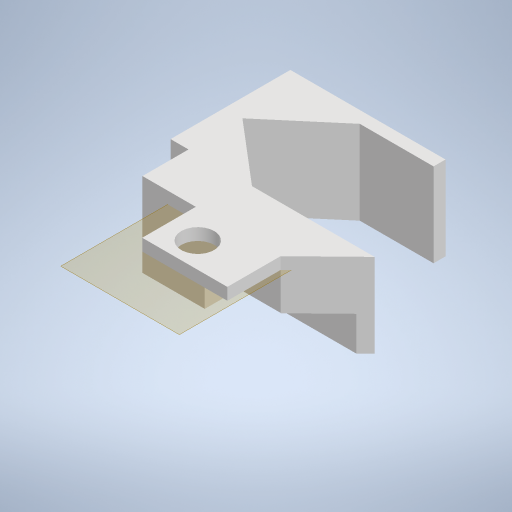
# Autodesk Inventor part: каретка
Saved by Autodesk Inventor 2024.2 (Build 282272000, 272)
## iProperties
Created: 2026-02-13
Part Number: каретка
Material: Типовые
Document SubType Name: Modeling
Designer: Service
Density: 1 g/cm^3
Appearance: По умолчанию
Author: Service
Autodesk Inventor part; units mm, degrees
ref_plane "YZ Plane" through (0, 0, 0) normal (1, 0, 0) x (0, 1, 0)
ref_plane "XZ Plane" through (0, 0, 0) normal (0, 1, 0) x (-1, 0, 0)
ref_plane "XY Plane" through (0, 0, 0) normal (0, 0, 1) x (1, 0, 0)
ref_plane "РабПлоскость1" through (-7.5749, -280.0826, 223.3085) normal (0, 1, 0) x (-1, 0, 0)
sketch "Эскиз1" plane through (-7.5749, -280.0826, 223.3085) normal (0, 1, 0) x (-1, 0, 0)
  line L0 (14.2093, 2.6473) -> (0, 2.6473)
  line L1 (0, 2.6473) -> (0, -6.2943)
  line L2 (0, -6.2943) -> (14.2093, -6.2943)
  line L3 (14.2093, -6.2943) -> (14.2093, 2.6473)
  line L4 (4.1714, -6.2943) -> (16.1714, -6.2943) projected
  line L5 (0, -6.2943) -> (0, -6.2338) projected
  circle A0 centre (9.1714, -1.5852) radius 2.75 projected
  line L6 (0, -6.2338) -> (-7.9567, -13.9803)
  line L7 (-7.9567, -13.9803) -> (14.2093, -13.9803)
  line L8 (14.2093, -13.9803) -> (14.2093, -6.2943)
  line L9 (-6.416, -12.4803) -> (14.2093, -12.4803)
  line L10 (12.7093, -6.2943) -> (12.7093, -12.4803)
  point P0 (-7.5749, -223.3085)
  point P1 (6.5045, -0.9144)
  point P2 (6.5045, -2.256)
  point P3 (0, -6.2338)
  point P4 (12.7093, -6.2943)
  dimension "d2" = 1.5
  dimension "d3" = 1.5
  constraints: 18 end point, 4 perpendicular, 4 point on line, 2 collinear, 2 horizontal, 2 parallel
  measures "d2" distance between parallel lines of L8 L10
  measures "d3" distance between parallel lines of L9 L7
extrude "Выдавливание1" add sketch "Эскиз1" along normal blind 2
extrude "Выдавливание2" add sketch "Эскиз1" against normal blind 12 contours L8 L9 L10 L2 | L8 L7 L6 L9
extrude "Выдавливание3" add sketch "Эскиз1" against normal blind 6.25 contours L1 L2 L10 L9 L6
sketch "Эскиз2" plane through (-7.5749, -278.0826, 223.3085) normal (0, 1, 0) x (1, 0, 0)
  line L0 (-14.2093, 13.9803) -> (7.9567, 13.9803) projected
  line L1 (-14.2093, 6.2943) -> (-23.1093, 6.2943)
  line L2 (-23.1093, 6.2943) -> (-23.1093, 13.9803)
  line L3 (-23.1093, 13.9803) -> (-14.2093, 13.9803)
  line L4 (-14.2093, 13.9803) -> (-14.2093, 6.2943)
  line L5 (-0.2093, 13.9803) -> (-23.1093, 13.9803)
  line L6 (-23.1093, 13.9803) -> (-23.1093, 33.9803)
  line L7 (-23.1093, 33.9803) -> (-0.2093, 33.9803)
  line L8 (-0.2093, 33.9803) -> (-0.2093, 13.9803)
  circle A0 centre (-9.2093, 22.9803) radius 9
  line L9 (-0.2093, 31.9803) -> (-23.1093, 31.9803)
  line L10 (-23.1093, 22.9803) -> (-12.5164, 31.9803)
  line L11 (-23.1093, 22.9803) -> (-12.5164, 13.9803)
  line L12 (-23.1093, 13.9803) -> (-26.1093, 13.9803)
  line L13 (-26.1093, 13.9803) -> (-26.1093, 33.9803)
  line L14 (-26.1093, 33.9803) -> (-23.1093, 33.9803)
  line L15 (-23.1093, 33.9803) -> (-23.1093, 13.9803)
  point P0 (7.5749, 223.3085)
  point P1 (-12.5164, 13.9803)
  point P2 (-23.1093, 33.9803)
  dimension "d13" = 20
  dimension "d14" = 18
  dimension "d15" = 2
  dimension "d16" = 8.9
  dimension "d17" = 22.9
  dimension "d18" = 3
  constraints: 30 end point, 7 point on line, 6 parallel, 4 horizontal, 4 tangent, 3 perpendicular, 1 centre point, 1 equal length
  measures "d13" distance of L5.end L6.end
  measures "d14" diameter of A0
  measures "d15" distance between parallel lines of L7 L9
  measures "d16" distance of L2.end L3.end
  measures "d17" distance between parallel lines of L6 L8
  measures "d18" distance between parallel lines of L15 L13
extrude "Выдавливание4" add sketch "Эскиз2" against normal up to surface (14 mm away) contours L3 L6 L11 L0 | L4 L1 L2 L3 | L12 L13 L14 L6 | L6 L9 L10 | L6 L7 L8 L9
